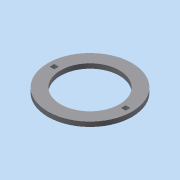
# Autodesk Inventor part: central
Saved by Autodesk Inventor 2015 (Build 190159000, 159)
## iProperties
Created: 2017-10-02
Part Number: central
Material: Generic
Document SubType Name: Modeling
Designer: macbook
Density: 1 g/cm^3
Appearance: Default
Author: macbook
Autodesk Inventor part; units mm, degrees
ref_plane "YZ Plane" through (0, 0, 0) normal (1, 0, 0) x (0, 1, 0)
ref_plane "XZ Plane" through (0, 0, 0) normal (0, 1, 0) x (-1, 0, 0)
ref_plane "XY Plane" through (0, 0, 0) normal (0, 0, 1) x (1, 0, 0)
sketch "Sketch1" plane through (0, 0, 0) normal (0, 0, 1) x (1, 0, 0)
  circle A0 centre (0, 0) radius 50
  circle A1 centre (0, 0) radius 35
  dimension "d0" = 100
  dimension "d1" = 70
  constraints: 2 centre point, 2 coincident
  measures "d0" diameter of A0
  measures "d1" diameter of A1
extrude "Extrusion1" add sketch "Sketch1" along normal blind 5.5
sketch "Sketch4" plane through (0, 0, 5.5) normal (0, 0, 1) x (1, 0, 0)
  line L0 (39.75, 2.75) -> (45.25, 2.75)
  line L1 (45.25, 2.75) -> (45.25, -2.75)
  line L2 (45.25, -2.75) -> (39.75, -2.75)
  line L3 (39.75, -2.75) -> (39.75, 2.75)
  line L4 (-39.75, -2.75) -> (-45.25, -2.75)
  line L5 (-45.25, -2.75) -> (-45.25, 2.75)
  line L6 (-45.25, 2.75) -> (-39.75, 2.75)
  line L7 (-39.75, 2.75) -> (-39.75, -2.75)
  point P0 (0, 0)
  dimension "d13" = 5.5
  dimension "d14" = 5.5
  dimension "d17" = 360
  constraints: 16 end point, 2 parallel, 1 horizontal, 1 perpendicular, 17 other
  measures "d13" distance of L1.end L2.end
  measures "d14" distance of L0.end L1.end
extrude "Extrusion3" cut sketch "Sketch4" against normal blind 10
body "Solid1"
